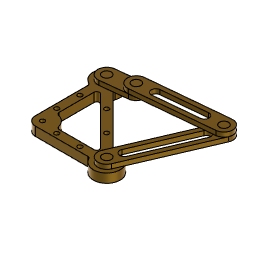
Ejercicio03jaalobuela (Autodesk Fusion 360 design; units mm, degrees)
Autodesk Fusion 360 part; units mm, degrees
sketch "Sketch1" plane through (0, 0, 0) normal (0, 0, 1) x (1, 0, 0)
  circle A0 centre (50, 150) radius 15
  circle A1 centre (50, 150) radius 5
  circle A2 centre (50, 120) radius 2.5
  circle A3 centre (50, 94) radius 2.5
  circle A4 centre (54, 74) radius 2.5
  circle A5 centre (74, 70) radius 2.5
  circle A6 centre (100, 70) radius 2.5
  circle A7 centre (130, 70) radius 5
  circle A8 centre (130, 70) radius 15
  circle A9 centre (101.7157, 98.2843) radius 2.5
  circle A10 centre (78.2843, 121.7157) radius 2.5
  line L0 (50, 150) -> (130, 70)
  line L1 (45, 150) -> (45, 65)
  line L2 (130, 65) -> (45, 65)
  line L3 (130, 70) -> (133.5355, 73.5355)
  line L4 (130, 70) -> (126.4645, 66.4645)
  line L5 (50, 150) -> (53.5355, 153.5355)
  line L6 (50, 150) -> (46.4645, 146.4645)
  line L7 (53.5355, 153.5355) -> (133.5355, 73.5355)
  line L8 (126.4645, 66.4645) -> (46.4645, 146.4645)
  line L9 (50, 94) -> (50, 93)
  arc A11 (68.9666, 75) -> (55, 88.9666) centre (54, 74) ccw
  line L10 (55, 150) -> (55, 88.9666)
  line L11 (130, 75) -> (68.9666, 75)
  circle A12 centre (-80, 70) radius 2.5
  circle A13 centre (-130, 120) radius 2.5
  circle A14 centre (-106, 70) radius 2.5
  line L12 (-130, 94) -> (-130, 93)
  line L13 (-67.1924, 80.1213) -> (-119.8787, 132.8076)
  circle A15 centre (-50, 70) radius 5
  arc A16 (-111.3751, 77.3333) -> (-122.6667, 88.6249) centre (-126, 74) ccw
  line L14 (-135, 133.8755) -> (-135, 75)
  circle A17 centre (-101.7157, 121.7157) radius 2.5
  circle A18 centre (-130, 94) radius 2.5
  line L15 (-115.0627, 142.1338) -> (-57.8662, 84.9373)
  circle A19 centre (-130, 150) radius 5
  circle A20 centre (-78.2843, 98.2843) radius 2.5
  line L16 (-66.1245, 65) -> (-125, 65)
  circle A21 centre (-126, 74) radius 2.5
  arc A22 (-115.7845, 145.2126) -> (-136.6667, 136.5629) centre (-130, 150) ccw
  line L17 (-125, 130.6863) -> (-125, 91.5499)
  arc A23 (-63.4371, 63.3333) -> (-54.7874, 84.2155) centre (-50, 70) ccw
  line L18 (-69.3137, 75) -> (-108.4501, 75)
  arc A24 (-135, 75) -> (-125, 65) centre (-125, 75) ccw
  arc A25 (-125, 91.5499) -> (-122.6667, 88.6249) centre (-122, 91.5499) ccw
  arc A26 (-111.3751, 77.3333) -> (-108.4501, 75) centre (-108.4501, 78) ccw
  arc A27 (-69.3137, 75) -> (-67.1924, 80.1213) centre (-69.3137, 78) ccw
  arc A28 (-57.8662, 84.9373) -> (-54.7874, 84.2155) centre (-55.7449, 87.0586) ccw
  arc A29 (-63.4371, 63.3333) -> (-66.1245, 65) centre (-66.1245, 62) ccw
  arc A30 (-135, 133.8755) -> (-136.6667, 136.5629) centre (-138, 133.8755) ccw
  arc A31 (-119.8787, 132.8076) -> (-125, 130.6863) centre (-122, 130.6863) ccw
  arc A32 (-115.7845, 145.2126) -> (-115.0627, 142.1338) centre (-112.9414, 144.2551) ccw
  dimension "d4" = 5
  dimension "d6" = 5
  dimension "d9" = 5
  dimension "d14" = 5
  dimension "d15" = 5
  dimension "d19" = 5
  dimension "d21" = 5
  dimension "d24" = 5
  dimension "d25" = 5
  dimension "d26" = 5
  dimension "d27" = 5
  dimension "d28" = 5
  dimension "d29" = 5
  dimension "d30" = 5
  dimension "d31" = 10
  dimension "d32" = 3
  dimension "d33" = 3
  dimension "d34" = 3
  dimension "d35" = 3
  dimension "d36" = 3
  dimension "d37" = 3
  dimension "d38" = 3
  dimension "d39" = 3
  constraint concentric A7 A8
  constraint coincident A0.centre A1.centre
  constraint coincident A7.centre A8.centre
  constraint coincident A1 L1.start
  constraint tangent A1 L1
  constraint vertical L1
  constraint coincident A1 L10.start
  constraint tangent A1 L10
  constraint coincident A7 L2.start
  constraint tangent A7 L2
  constraint perpendicular L1 L2
  constraint coincident A7 L11.start
  constraint tangent A7 L11
  constraint perpendicular L1 L11
  constraint coincident A7 L3.end
  constraint perpendicular L0 L3
  constraint coincident A7 L4.end
  constraint perpendicular L0 L4
  constraint coincident A1 L5.end
  constraint perpendicular L0 L5
  constraint coincident A1 L6.end
  constraint perpendicular L0 L6
  constraint tangent A7 L7
  constraint tangent A1 L8
  constraint coincident A3.centre L9.start
  constraint parallel L1 L9
  constraint concentric A15 A23
  constraint tangent L14 A19
  constraint vertical L14
  constraint tangent A15 L16
  constraint perpendicular L14 L16
  constraint tangent A15 L15
  constraint tangent L13 A19
  constraint coincident L12.start A18.centre
  constraint parallel L12 L14
  constraint tangent L14 A24
  constraint tangent L16 A24
  constraint tangent A16 A25
  constraint tangent L17 A25
  constraint tangent A16 A26
  constraint tangent L18 A26
  constraint tangent L18 A27
  constraint tangent L13 A27
  constraint tangent A23 A28
  constraint tangent L15 A28
  constraint tangent A23 A29
  constraint tangent L16 A29
  constraint tangent A22 A30
  constraint tangent L14 A30
  constraint tangent L17 A31
  constraint tangent L13 A31
  constraint tangent A22 A32
  constraint tangent L15 A32
  measures "d4" diameter of A2
  measures "d6" diameter of A3
  measures "d9" diameter of A4
  measures "d14" diameter of A5
  measures "d15" diameter of A6
  measures "d19" diameter of A9
  measures "d21" diameter of A10
  measures "d24" diameter of A13
  measures "d25" diameter of A18
  measures "d26" diameter of A21
  measures "d27" diameter of A14
  measures "d28" diameter of A12
  measures "d29" diameter of A20
  measures "d30" diameter of A17
  measures "d31" radius of A24
  measures "d32" radius of A25
  measures "d33" radius of A26
  measures "d34" radius of A27
  measures "d35" radius of A28
  measures "d36" radius of A29
  measures "d37" radius of A30
  measures "d38" radius of A31
  measures "d39" radius of A32
extrude "Extrude1" add sketch "Sketch1" along normal blind 10 contours L14 L15 L16 A22 A23 A24 A28 A29 A30 A32 makes body 1
sketch "Sketch2" plane through (0, 0, 0) normal (0, 0, 1) x (1, 0, 0)
  line L0 (25, 145) -> (55, 145)
  line L1 (55, 125) -> (25, 125)
  circle A0 centre (25, 135) radius 5
  circle A1 centre (55, 135) radius 5
  arc A2 (25, 145) -> (25, 125) centre (25, 135) ccw
  arc A3 (55, 125) -> (55, 145) centre (55, 135) ccw
  dimension "d48" = 20
  dimension "d49" = 20
  dimension "d50" = 10
  dimension "d51" = 10
  constraint tangent L0 A3
  constraint tangent L1 A2
  constraint concentric A1 A3
  measures "d48" diameter of A2
  measures "d49" diameter of A3
  measures "d50" diameter of A0
  measures "d51" diameter of A1
sketch "Sketch3" plane through (0, 0, 0) normal (0, 0, 1) x (1, 0, 0)
extrude "Extrude3" add sketch "Sketch2" along normal blind 5 separate body makes body 2
sketch "Sketch4" plane through (0, 0, 0) normal (0, 0, 1) x (1, 0, 0)
  line L0 (-80, 210) -> (20, 210)
  line L1 (20, 190) -> (-80, 190)
  circle A0 centre (-80, 200) radius 5
  circle A1 centre (20, 200) radius 5
  arc A2 (20, 190) -> (20, 210) centre (20, 200) ccw
  arc A3 (-80, 210) -> (-80, 190) centre (-80, 200) ccw
  arc A4 (140, 210) -> (140, 190) centre (140, 200) ccw
  circle A5 centre (230, 200) radius 5
  circle A6 centre (140, 200) radius 5
  arc A7 (230, 190) -> (230, 210) centre (230, 200) ccw
  line L2 (20, 200) -> (5, 200)
  line L3 (-65, 205) -> (5, 205)
  line L4 (5, 195) -> (-65, 195)
  arc A8 (-65, 205) -> (-65, 195) centre (-65, 200) ccw
  arc A9 (5, 195) -> (5, 205) centre (5, 200) ccw
  line L5 (140, 190) -> (230, 190)
  line L6 (140, 210) -> (230, 210)
  line L7 (210, 195) -> (160.0189, 195)
  line L8 (160.0189, 205) -> (210, 205)
  arc A10 (160.0189, 205) -> (160.0189, 195) centre (160.0189, 200) ccw
  arc A11 (210, 195) -> (210, 205) centre (210, 200) ccw
  dimension "d54" = 100
  dimension "d55" = 20
  dimension "d56" = 10
  dimension "d57" = 10
  dimension "d59" = 20
  dimension "d60" = 10
  dimension "d61" = 10
  dimension "d63" = 15
  dimension "d64" = 10
  dimension "d65" = 10
  dimension "d69" = 10
  dimension "d71" = 10
  constraint horizontal L0
  constraint horizontal L1
  constraint concentric A0 A3
  constraint concentric A1 A2
  constraint concentric A4 A6
  constraint concentric A5 A7
  constraint coincident A1.centre A2.centre
  constraint parallel L0 L2
  constraint coincident L2.end A9.centre
  constraint tangent L3 A9
  constraint tangent L4 A8
  constraint parallel L2 L4
  constraint horizontal L5
  constraint horizontal L6
  constraint tangent L7 A10
  constraint tangent L8 A11
  measures "d54" distance of L0.start L0.end
  measures "d55" distance of L0.start L1.end
  measures "d56" diameter of A0
  measures "d57" diameter of A1
  measures "d59" distance of A4.end A4.start
  measures "d60" diameter of A6
  measures "d61" diameter of A5
  measures "d63" distance of A1.centre L2.end
  measures "d64" diameter of A8
  measures "d65" diameter of A9
  measures "d69" diameter of A10
  measures "d71" diameter of A11
extrude "Extrude4" add sketch "Sketch4" along normal blind 5 separate body contours L0 L1 A2 A3 makes body 3
extrude "Extrude5" add sketch "Sketch4" along normal blind 5 separate body contours A4 A7 L5 L6 makes body 4
cylinder "CylinderPrimitive1" add diameter 10 height 10 placed x (1, 0, 0) y (0, 1, 0) z (0, 0, 1) at (20, 55, 0) separate body makes body 5
cylinder "CylinderPrimitive2" add diameter 10 height 15 placed x (1, 0, 0) y (0, 1, 0) z (0, 0, 1) at (-5, 10, 0) separate body makes body 6
move_body "Move1" bodies 6 to x (1, 0, 0) y (0, 1, 0) z (0, 0, 1) at (-45, 60, 0)
move_body "Move2" bodies 6 to x (1, 0, 0) y (0, 1, 0) z (0, 0, 1) at (0, 0, 20)
copy_body "CopyPasteBodies1" bodies 6 makes body 7
move_body "Move3" bodies 7 to x (1, 0, 0) y (0, 1, 0) z (0, 0, 1) at (-80, 80, -20)
move_body "Move4" bodies 6 to x (1, 0, 0) y (0, 1, 0) z (0, 0, 1) at (0, 0, -20)
copy_body "Body->Comp1" bodies 1 removing the originals makes body 8 in component "Component"
copy_body "Body->Comp2" bodies 3 removing the originals makes body 9 in component "Component'"
copy_body "Body->Comp3" bodies 2 removing the originals makes body 10 in component "Component''"
copy_body "Body->Comp4" bodies 4 removing the originals makes body 11 in component "Component'''"
move_body "Move5" bodies 7 6 to x (1, 0, 0) y (0, 1, 0) z (0, 0, 1) at (0, 0, 50)
copy_body "CopyPasteBodies2" bodies 5 makes body 12
move_body "Move6" bodies 12 to x (1, 0, 0) y (0, 1, 0) z (0, 0, 1) at (75, 0, 0)
copy_body "Body->Comp5" bodies 7 removing the originals makes body 13 in component "Component''''"
copy_body "Body->Comp6" bodies 6 removing the originals makes body 14 in component "Component'''''"
copy_body "Body->Comp7" bodies 12 removing the originals makes body 15 in component "Component''''''"
copy_body "Body->Comp8" bodies 5 removing the originals makes body 16 in component "Component'''''''"
component "Component" placed x (1, 0, 0) y (0, 1, 0) z (0, 0, 1) at (0, 0, 0)
component "Component'" placed x (0.394077, 0.919077, 0) y (-0.919077, 0.394077, 0) z (0, 0, 1) at (165.3416, 64.7107, 10)
component "Component''" placed x (0.995132, 0.098552, 0) y (-0.098552, 0.995132, 0) z (0, 0, 1) at (-141.5738, 13.1934, 10)
component "Component'''" placed x (0.995042, 0.099458, 0) y (-0.099458, 0.995042, 0) z (0, 0, 1) at (-219.5604, -59.9759, 15)
component "Component''''" placed x (1, 0, 0) y (0, 1, 0) z (0, 0, 1) at (0, 0, -50)
component "Component'''''" placed x (1, 0, 0) y (0, 1, 0) z (0, 0, 1) at (0, 0, -50)
component "Component''''''" placed x (0.995132, 0.098552, 0) y (-0.098552, 0.995132, 0) z (0, 0, 1) at (-189.2632, 88.8619, 10)
component "Component'''''''" placed x (0.995042, 0.099458, 0) y (-0.099458, 0.995042, 0) z (0, 0, 1) at (-25.023, 105.1913, 10)
